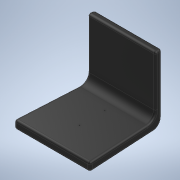
# Autodesk Inventor part: chair
Saved by Autodesk Inventor 2022 (Build 260153000, 153)
## iProperties
Created: 2021-12-06
Part Number: chair
Material: Generic
Document SubType Name: Modeling
Designer: Vedic
Density: 1 g/cm^3
Appearance: Default
Author: Vedic
Autodesk Inventor part; units mm, degrees
ref_plane "YZ Plane" through (0, 0, 0) normal (1, 0, 0) x (0, 1, 0)
ref_plane "XZ Plane" through (0, 0, 0) normal (0, 1, 0) x (-1, 0, 0)
ref_plane "XY Plane" through (0, 0, 0) normal (0, 0, 1) x (1, 0, 0)
sketch "Sketch1" plane through (0, 0, 0) normal (0, 1, 0) x (-1, 0, 0)
  line L0 (200.011876, 171.42375) -> (-257.188124, 171.42375)
  line L1 (-257.188124, 171.42375) -> (-231.788124, -285.77625)
  line L2 (-231.788124, -285.77625) -> (174.611876, -285.77625)
  line L3 (174.611876, -285.77625) -> (200.011876, 171.42375)
  point P0 (0, 0)
  dimension "d0" = 457.2
  dimension "d1" = 457.2
  dimension "d2" = 406.4
  constraints: 8 end point, 1 equal length, 1 horizontal, 1 parallel
  measures "d0" distance of L0.start L0.end
  measures "d1" distance between parallel lines of L2 L0
  measures "d2" distance of L1.end L2.end
extrude "Extrusion1" add sketch "Sketch1" along normal blind 50.8
sketch "Sketch2" plane through (0, 50.8, 0) normal (0, 1, 0) x (1, 0, 0)
  line L0 (231.788124, 285.77625) -> (-174.611876, 285.77625)
  line L1 (-174.611876, 285.77625) -> (-176.728543, 247.67625)
  line L2 (-174.611876, 285.77625) -> (-200.011876, -171.42375)
  line L3 (-176.728543, 247.67625) -> (233.904791, 247.67625)
  line L4 (257.188124, -171.42375) -> (231.788124, 285.77625)
  line L5 (233.904791, 247.67625) -> (231.788124, 285.77625)
  line L6 (231.788124, 285.77625) -> (-174.611876, 285.77625)
  point P0 (0, 0)
  dimension "d5" = 38.1
  constraints: 8 end point, 2 point on line, 1 collinear, 1 horizontal
  measures "d5" distance between parallel lines of L0 L3
extrude "Extrusion2" add sketch "Sketch2" along normal blind 355.6
fillet "Fillet1" radius 50.8 1 edges at (28.5881, 50.8, -247.6762)
fillet "Fillet2" radius 12.7 4 edges at (28.5881, 0, 171.4238) (28.5881, 50.8, 171.4238) (28.5881, 406.4, -247.6762) (28.5881, 406.4, -285.7762)
fillet "Fillet3" radius 50.8 1 edges at (28.5881, 0, -285.7762)
fillet "Fillet4" radius 12.7 20 edges at (232.6147, 14.879, -270.8973) (231.7881, 222.25, -285.7762) (231.9948, 402.6803, -282.0565) (232.8465, 406.4, -266.7262) (233.6981, 402.6803, -251.396) (233.9048, 247.65, -247.6762) (234.7314, 65.679, -232.7973) (246.6048, 50.8, -19.0762) (256.9815, 3.7197, 167.704) (245.5465, 0, -38.1262) (-199.8052, 3.7197, 167.704) (-188.3702, 0, -38.1262) (-175.4385, 14.879, -270.8973) (-174.6119, 222.25, -285.7762) (-174.8185, 402.6803, -282.0565) (-175.6702, 406.4, -266.7262) (-176.5219, 402.6803, -251.396) (-176.7285, 247.65, -247.6762) (-177.5552, 65.679, -232.7973) (-189.4285, 50.8, -19.0762)
sketch "Sketch3" plane through (0, 50.8, 0) normal (0, 1, 0) x (1, 0, 0)
  line L0 (221.890763, 234.97625) -> (-164.714514, 234.97625)
  line L1 (28.588124, 234.97625) -> (28.588124, -158.72375) construction
  line L2 (-186.586737, -158.72375) -> (243.762985, -158.72375)
  circle A0 centre (28.588124, -6.32375) radius 3.175
  circle A1 centre (28.588124, 146.07625) radius 3.175
  point P0 (0, 0)
  dimension "d13" = 6.35
  dimension "d14" = 152.4
  dimension "d15" = 152.4
  constraints: 2 centre point, 2 end point, 2 midpoint, 2 point on line, 1 equal radius
  measures "d13" diameter of A1
  measures "d14" distance of A0.centre A1.centre
  measures "d15" distance from line of L2 A0.centre
extrude "Extrusion3" cut sketch "Sketch3" against normal through all
body "Solid1"
